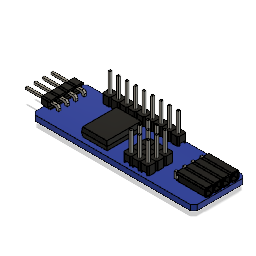
IOExpanderPCF8574T (Autodesk Fusion 360 design; units mm, degrees)
Autodesk Fusion 360 part; units mm, degrees
note: some values were not read from the file. Set by a fixed rule: which sketch regions a step uses.
sketch "Sketch1" plane through (0, 0, 0) normal (0, 1, 0) x (1, 0, 0) in component "PCB"
  line L0 (0, 0) -> (48.25, 0)
  line L1 (48.25, 0) -> (48.25, -15.6)
  line L2 (48.25, -15.6) -> (0, -15.6)
  line L3 (0, -15.6) -> (0, 0)
  dimension "d1" = 48.25
  dimension "d2" = 15.6
  dimension "d35" = 0
  dimension "d36" = 0
  dimension "d37" = 0
  dimension "d38" = 0
  measures "d2" distance of L0.start
extrude "Extrude1" add sketch "Sketch1" along normal blind 1.62 makes body 1 in component "PCB"
chamfer "Chamfer1" distance 1 angle 45 4 edges at (0, 0.81, 15.6) (48.25, 0.81, 15.6) (48.25, 0.81, 0) (0, 0.81, 0) on bodies 1 in component "PCB"
sketch "Sketch1 (1)" plane through (0, 1.62, 0) normal (0, 1, 0) x (-1, 0, 0) in component "PCB"
  line L0 (-1, 0) -> (0, 1)
  line L1 (0, 1) -> (0, 14.6)
  line L2 (0, 14.6) -> (-1, 15.6)
  line L3 (-1, 15.6) -> (-47.25, 15.6)
  line L4 (-47.25, 15.6) -> (-48.25, 14.6)
  line L5 (-48.25, 14.6) -> (-48.25, 1)
  line L6 (-48.25, 1) -> (-47.25, 0)
  line L7 (-47.25, 0) -> (-1, 0)
  line L8 (-3.3, 0) -> (-3.3, 3.3) construction
  line L9 (0, 3.3) -> (-3.3, 3.3) construction
  line L10 (-3.3, 3.3) -> (-3.3, 5.84) construction
  line L11 (-3.3, 5.84) -> (-3.3, 8.38) construction
  line L12 (-3.3, 8.38) -> (-3.3, 10.92) construction
  line L13 (0, 1.3) -> (-9, 1.3) construction
  line L14 (-9, 0) -> (-9, 1.3) construction
  line L15 (-9, 1.3) -> (-11.54, 1.3) construction
  line L16 (-11.54, 1.3) -> (-14.08, 1.3) construction
  line L17 (-14.08, 1.3) -> (-16.62, 1.3) construction
  line L18 (-16.62, 1.3) -> (-19.16, 1.3) construction
  line L19 (-19.16, 1.3) -> (-21.7, 1.3) construction
  line L20 (-21.7, 1.3) -> (-24.24, 1.3) construction
  line L21 (-24.24, 1.3) -> (-26.78, 1.3) construction
  line L22 (-26.78, 1.3) -> (-29.32, 1.3) construction
  line L23 (-38.35, 0) -> (-38.35, 3.3) construction
  line L24 (-48.25, 3.3) -> (-38.35, 3.3) construction
  line L25 (-38.35, 3.3) -> (-38.35, 5.84) construction
  line L26 (-38.35, 5.84) -> (-38.35, 8.38) construction
  line L27 (-38.35, 8.38) -> (-38.35, 10.92) construction
  line L28 (-32.45, 15.6) -> (-32.45, 13.4) construction
  line L29 (-48.25, 13.4) -> (-32.45, 13.4) construction
  line L30 (-32.45, 13.4) -> (-29.91, 13.4) construction
  line L31 (-29.91, 13.4) -> (-27.37, 13.4) construction
  line L32 (-27.37, 13.4) -> (-27.37, 10.86) construction
  line L33 (-27.37, 10.86) -> (-29.91, 10.86) construction
  line L34 (-29.91, 10.86) -> (-32.45, 10.86) construction
  line L35 (-32.45, 10.86) -> (-32.45, 8.32) construction
  line L36 (-32.45, 8.32) -> (-29.91, 8.32) construction
  line L37 (-29.91, 8.32) -> (-27.37, 8.32) construction
  dimension "d6" = 3.3
  dimension "d7" = 3.3
  dimension "d8" = 2.54
  dimension "d9" = 9
  dimension "d10" = 1.3
  dimension "d11" = 2.54
  dimension "d12" = 3.3
  dimension "d13" = 9.9
  dimension "d14" = 2.54
  dimension "d15" = 2.2
  dimension "d16" = 15.8
  dimension "d17" = 2.54
  measures "d12" distance of origin
hole "Hole1" at (27.37, 1.62, 8.32) at (29.91, 1.62, 8.32) at (32.45, 1.62, 8.32) at (32.45, 1.62, 10.86) at (29.91, 1.62, 10.86) at (27.37, 1.62, 10.86) at (27.37, 1.62, 13.4) at (29.91, 1.62, 13.4) at (32.45, 1.62, 13.4) at (38.35, 1.62, 10.92) at (38.35, 1.62, 8.38) at (38.35, 1.62, 5.84) at (38.35, 1.62, 3.3) at (29.32, 1.62, 1.3) at (26.78, 1.62, 1.3) at (24.24, 1.62, 1.3) at (21.7, 1.62, 1.3) at (19.16, 1.62, 1.3) at (16.62, 1.62, 1.3) at (14.08, 1.62, 1.3) at (11.54, 1.62, 1.3) at (9, 1.62, 1.3) at (3.3, 1.62, 10.92) at (3.3, 1.62, 8.38) at (3.3, 1.62, 5.84) at (3.3, 1.62, 3.3) direction (0, -1, 0) diameter 0.635 depth 9.6 tip angle 180 bodies 1 in component "PCB"
sketch "Sketch1 (2)" plane through (0, 0, 0) normal (0, 1, 0) x (1, 0, 0) in component "Pin"
  line L0 (0, 0) -> (5.08, 0)
  line L1 (5.08, 0) -> (5.08, -0.635)
  line L2 (5.08, -0.635) -> (0.635, -0.635)
  line L3 (0, -5.08) -> (0, 0)
  line L4 (0.635, -0.635) -> (0.635, -5.08)
  line L5 (0, -5.08) -> (0.635, -5.08)
  dimension "d3_1" = 5.08
  dimension "d29" = 0.635
  dimension "d30" = 5.08
  measures "d3_1" distance of L0.start
  measures "d30" distance of L0.start
extrude "Extrude1'" add sketch "Sketch1 (2)" along normal blind 0.635 separate body makes body 2 in component "Pin"
chamfer "Chamfer1'" distance 0.1905 angle 45 4 edges at (0.3175, 0.635, 5.08) (0.3175, 0, 5.08) (0.635, 0.3175, 5.08) (0, 0.3175, 5.08) on bodies 2 in component "Pin"
sketch "Sketch1 (3)" plane through (0, 0, 0) normal (0, 1, 0) x (1, 0, 0) in component "Plastic"
  line L0 (0, -0.3175) -> (2.159, -0.3175)
  line L1 (2.159, -1.0795) -> (2.159, 0.4445)
  line L2 (2.159, 0.4445) -> (2.1592, 0.9525) construction
  line L3 (2.159, -1.0795) -> (2.159, -1.5875) construction
  line L4 (2.159, 0.4445) -> (1.524, 0.4445)
  line L5 (2.159, -1.0795) -> (1.524, -1.0795)
  line L6 (1.524, -1.0795) -> (1.524, -1.5875)
  line L7 (1.524, 0.4445) -> (1.524, 0.9525)
  line L8 (1.524, 0.9525) -> (10.16, 0.9525)
  line L9 (10.16, 0.9525) -> (10.16, -1.5875)
  line L10 (1.524, -1.5875) -> (10.16, -1.5875)
  line L11 (0, 0) -> (0, -0.635) construction
  dimension "d7_1" = 2.159
  dimension "d8_1" = 1.524
  dimension "d9_1" = 0.508
  dimension "d11_1" = 0.635
  dimension "d12_1" = 8.636
  measures "d7_1" distance of L11.start
extrude "Extrude1''" add sketch "Sketch1 (3)" along normal mid plane 2.54 from surface at 0.3175 separate body makes body 3 in component "Plastic"
chamfer "Chamfer1''" distance 0.4 angle 45 4 edges at (5.842, 1.5875, -0.9525) (5.842, -0.9525, -0.9525) (5.842, 1.5875, 1.5875) (5.842, -0.9525, 1.5875) on bodies 3 in component "Plastic"
sketch "Sketch1 (4)" plane through (0, 0, 0) normal (0, 0, 1) x (1, 0, 0) in component "Pins bent female v2"
  line L0 (0, 0.3175) -> (0, 14)
other "PathPattern1" in component "Header"
sketch "Sketch1 (1) (2)" plane through (10.16, 0, 0) normal (1, 0, 0) x (0, 0, -1) in component "Plastic"
  line L0 (-1.5875, -0.5525) -> (-1.1875, -0.9525)
  line L1 (-1.1875, -0.9525) -> (0.5525, -0.9525)
  line L2 (0.5525, -0.9525) -> (0.9525, -0.5525)
  line L3 (0.9525, -0.5525) -> (0.9525, 1.1875)
  line L4 (0.9525, 1.1875) -> (0.5525, 1.5875)
  line L5 (0.5525, 1.5875) -> (-1.1875, 1.5875)
  line L6 (-1.1875, 1.5875) -> (-1.5875, 1.1875)
  line L7 (-1.5875, 1.1875) -> (-1.5875, -0.5525)
  line L8 (0.9525, 0.3175) -> (-0.3175, 0.3175) construction
  line L9 (-0.3175, 1.5875) -> (-0.3175, 0.3175) construction
  line L10 (-0.3175, 0.635) -> (0, 0.635)
  line L11 (0, 0.3175) -> (0, 0)
  line L12 (0, 0) -> (-0.635, 0)
  line L13 (-0.635, 0) -> (-0.635, 0.635)
  line L14 (0, 0.635) -> (0, 0.3175)
  line L15 (-0.635, 0.635) -> (-0.3175, 0.635)
  dimension "d24" = 0.635
  dimension "d25" = 0.635
  measures "d25" distance of L11.end
extrude "Extrude1'''" cut sketch "Sketch1 (1) (2)" against normal blind 5.5 contours L10 L11 L12 L13 L14 L15 bodies 3 in component "Plastic"
chamfer "Chamfer1'''" distance 0.6 angle 45 4 edges at (10.16, 0, 0.3175) (10.16, 0.3175, 0) (10.16, 0.635, 0.3175) (10.16, 0.3175, 0.635) on bodies 3 in component "Plastic"
sketch "Sketch1 (5)" plane through (0, 0, 0) normal (0, 1, 0) x (1, 0, 0) in component "Pin (1)"
  line L0 (11.684, 0) -> (11.684, -0.635)
  line L1 (0, -0.3175) -> (1.524, -0.3175) construction
  line L2 (1.524, 0) -> (1.524, -4.572)
  line L3 (1.524, 0) -> (11.684, 0)
  line L4 (11.684, -0.635) -> (2.159, -0.635)
  line L5 (2.159, -0.635) -> (1.524, -0.635) construction
  line L6 (2.159, -0.635) -> (2.159, -4.572)
  line L7 (2.159, -4.572) -> (1.524, -4.572)
  dimension "d3_2" = 11.684
  dimension "d19_2" = 1.524
  dimension "d20_2" = 0.635
  dimension "d21_1" = 4.572
  measures "d3_2" distance of origin
  measures "d19_2" distance of origin
extrude "Extrude1''''" add sketch "Sketch1 (5)" along normal blind 0.635 separate body makes body 4 in component "Pin (1)"
fillet "Fillet1" radius 0.75 2 edges at (2.159, 0.3175, 0.635) (1.524, 0.3175, 0) on bodies 4 in component "Pin (1)"
chamfer "Chamfer1''''" distance 0.1905 angle 45 8 edges at (11.684, 0.3175, 0.635) (11.684, 0.635, 0.3175) (11.684, 0.3175, 0) (11.684, 0, 0.3175) (2.159, 0.3175, 4.572) (1.524, 0.3175, 4.572) (1.8415, 0.635, 4.572) (1.8415, 0, 4.572) on bodies 4 in component "Pin (1)"
sketch "Sketch1 (6)" plane through (0, 0, 0) normal (0, 0, 1) x (1, 0, 0) in component "Pins bent male v10"
  line L0 (0, 0.3175) -> (0, 14)
  line L1 (1.7145, 0.1905) -> (1.7145, 0.4445)
  line L2 (1.7145, 0.3175) -> (0, 0.3175) construction
sketch "Sketch1 (7)" plane through (0, 0, 0) normal (0, 1, 0) x (1, 0, 0) in component "Plastic (1)"
  line L0 (0, -0.3175) -> (3.81, -0.3175)
  line L1 (3.81, -1.0795) -> (3.81, 0.4445)
  line L2 (3.81, 0.4445) -> (3.81, 0.9525) construction
  line L3 (3.81, -1.0795) -> (3.81, -1.5875) construction
  line L4 (3.81, 0.4445) -> (3.175, 0.4445)
  line L5 (3.81, -1.0795) -> (3.175, -1.0795)
  line L6 (3.175, -1.0795) -> (3.175, -1.5875)
  line L7 (3.175, 0.4445) -> (3.175, 0.9525)
  line L8 (3.175, 0.9525) -> (5.715, 0.9525)
  line L9 (5.715, 0.9525) -> (5.715, -1.5875)
  line L10 (3.175, -1.5875) -> (5.715, -1.5875)
  dimension "d7_2" = 3.81
  dimension "d8_2" = 1.524
  dimension "d9_2" = 0.508
  dimension "d11_2" = 0.635
  dimension "d12_2" = 2.54
  measures "d7_2" distance of origin
extrude "Extrude1'''''" add sketch "Sketch1 (7)" along normal mid plane 2.54 from surface at 0.3175 separate body makes body 5 in component "Plastic (1)"
chamfer "Chamfer1'''''" distance 0.4 angle 45 4 edges at (4.445, 1.5875, -0.9525) (4.445, -0.9525, -0.9525) (4.445, 1.5875, 1.5875) (4.445, -0.9525, 1.5875) on bodies 5 in component "Plastic (1)"
other "PathPattern2" in component "Pins bent male v10"
sketch "Sketch1 (8)" plane through (0, 0, 0) normal (0, 1, 0) x (1, 0, 0) in component "Pin (2)"
  line L0 (0, 0) -> (11.684, 0)
  line L1 (11.684, 0) -> (11.684, -0.635)
  line L2 (11.684, -0.635) -> (0, -0.635)
  line L3 (0, -0.635) -> (0, 0)
  dimension "d2_1" = 0.635
  dimension "d3_3" = 11.684
  measures "d3_3" distance of L0.start
extrude "Extrude1''''''" add sketch "Sketch1 (8)" along normal blind 0.635 separate body makes body 6 in component "Pin (2)"
chamfer "Chamfer1''''''" distance 0.1905 angle 45 8 edges at (0, 0.3175, 0.635) (0, 0.635, 0.3175) (0, 0.3175, 0) (0, 0, 0.3175) (11.684, 0.635, 0.3175) (11.684, 0.3175, 0) (11.684, 0, 0.3175) (11.684, 0.3175, 0.635) on bodies 6 in component "Pin (2)"
sketch "Sketch1 (9)" plane through (0, 0, 0) normal (0, 1, 0) x (1, 0, 0) in component "Plastic (2)"
  line L0 (0, -0.4445) -> (0, -0.1905)
  line L1 (0, -0.3175) -> (3.81, -0.3175)
  line L2 (3.81, -1.0795) -> (3.81, 0.4445)
  line L3 (0.1905, 0) -> (11.4935, 0) construction
  line L4 (3.81, 0.4445) -> (3.81, 0.9525) construction
  line L5 (3.81, -1.0795) -> (3.81, -1.5875) construction
  line L6 (3.81, 0.4445) -> (3.175, 0.4445)
  line L7 (3.81, -1.0795) -> (3.175, -1.0795)
  line L8 (3.175, -1.0795) -> (3.175, -1.5875)
  line L9 (3.175, 0.4445) -> (3.175, 0.9525)
  line L10 (3.175, 0.9525) -> (5.715, 0.9525)
  line L11 (5.715, 0.9525) -> (5.715, -1.5875)
  line L12 (3.175, -1.5875) -> (5.715, -1.5875)
  dimension "d7_3" = 3.81
  dimension "d8_3" = 1.524
  dimension "d9_3" = 0.508
  dimension "d11_3" = 0.635
  dimension "d12_3" = 2.54
  measures "d7_3" distance of origin
extrude "Extrude1'''''''" add sketch "Sketch1 (9)" along normal mid plane 2.54 from surface at 0.3175 separate body makes body 7 in component "Plastic (2)"
chamfer "Chamfer1'''''''" distance 0.4 angle 45 4 edges at (4.445, 1.5875, -0.9525) (4.445, -0.9525, -0.9525) (4.445, 1.5875, 1.5875) (4.445, -0.9525, 1.5875) on bodies 7 in component "Plastic (2)"
sketch "Sketch1 (10)" plane through (0, 0, 0) normal (0, 0, 1) x (1, 0, 0) in component "Pins straight male v6"
  line L0 (0, 0.1905) -> (0, 0.4445)
  line L1 (0, 0.3175) -> (0, 14)
other "PathPattern1'" in component "Header (2)"
sketch "Sketch1 (11)" plane through (0, 0, 0) normal (0, 1, 0) x (1, 0, 0) in component "Pin (3)"
  line L0 (0, 0) -> (11.684, 0)
  line L1 (11.684, 0) -> (11.684, -0.635)
  line L2 (11.684, -0.635) -> (0, -0.635)
  line L3 (0, -0.635) -> (0, 0)
  dimension "d2_2" = 0.635
  dimension "d3_4" = 11.684
  dimension "d31" = 0
  dimension "d32" = 0
  dimension "d33" = 0
  dimension "d34" = 0
  measures "d3_4" distance of L0.start
extrude "Extrude1''''''''" add sketch "Sketch1 (11)" along normal blind 0.635 separate body makes body 8 in component "Pin (3)"
chamfer "Chamfer1''''''''" distance 0.1905 angle 45 8 edges at (0, 0.3175, 0.635) (0, 0.635, 0.3175) (0, 0.3175, 0) (0, 0, 0.3175) (11.684, 0.635, 0.3175) (11.684, 0.3175, 0) (11.684, 0, 0.3175) (11.684, 0.3175, 0.635) on bodies 8 in component "Pin (3)"
sketch "Sketch1 (12)" plane through (0, 0, 0) normal (0, 1, 0) x (1, 0, 0) in component "Plastic (3)"
  line L0 (0, -0.4445) -> (0, -0.1905)
  line L1 (0, -0.3175) -> (3.81, -0.3175)
  line L2 (3.81, -1.0795) -> (3.81, 0.4445)
  line L3 (0.1905, 0) -> (11.4935, 0) construction
  line L4 (3.81, 0.4445) -> (3.81, 0.9525) construction
  line L5 (3.81, -1.0795) -> (3.81, -1.5875) construction
  line L6 (3.81, 0.4445) -> (3.175, 0.4445)
  line L7 (3.81, -1.0795) -> (3.175, -1.0795)
  line L8 (3.175, -1.0795) -> (3.175, -1.5875)
  line L9 (3.175, 0.4445) -> (3.175, 0.9525)
  line L10 (3.175, 0.9525) -> (5.715, 0.9525)
  line L11 (5.715, 0.9525) -> (5.715, -1.5875)
  line L12 (3.175, -1.5875) -> (5.715, -1.5875)
  dimension "d7_4" = 3.81
  dimension "d8_4" = 1.524
  dimension "d9_4" = 0.508
  dimension "d11_4" = 0.635
  dimension "d12_4" = 2.54
  measures "d7_4" distance of origin
extrude "Extrude1'''''''''" add sketch "Sketch1 (12)" along normal mid plane 2.54 from surface at 0.3175 separate body makes body 9 in component "Plastic (3)"
chamfer "Chamfer1'''''''''" distance 0.4 angle 45 4 edges at (4.445, 1.5875, -0.9525) (4.445, -0.9525, -0.9525) (4.445, 1.5875, 1.5875) (4.445, -0.9525, 1.5875) on bodies 9 in component "Plastic (3)"
sketch "Sketch1 (13)" plane through (0, 0, 0) normal (0, 0, 1) x (1, 0, 0) in component "Pins straight male v7"
  line L0 (0, 0.1905) -> (0, 0.4445)
  line L1 (0, 0.3175) -> (0, 14)
other "PathPattern1''" in component "Header (3)"
sketch "Sketch1 (14)" plane through (0, 1.62, 0) normal (0, 1, 0) x (-1, 0, 0) in component "Chip"
  circle A0 centre (-3.3, 5.84) radius 0.3175
  circle A1 centre (-3.3, 10.92) radius 0.3175
  circle A2 centre (-11.54, 1.3) radius 0.3175
  circle A3 centre (-16.62, 1.3) radius 0.3175
  circle A4 centre (-21.7, 1.3) radius 0.3175
  circle A5 centre (-26.78, 1.3) radius 0.3175
  circle A6 centre (-38.35, 3.3) radius 0.3175
  circle A7 centre (-38.35, 8.38) radius 0.3175
  circle A8 centre (-32.45, 13.4) radius 0.3175
  circle A9 centre (-27.37, 13.4) radius 0.3175
  circle A10 centre (-29.91, 10.86) radius 0.3175
  circle A11 centre (-32.45, 8.32) radius 0.3175
  circle A12 centre (-27.37, 8.32) radius 0.3175
  circle A13 centre (-29.91, 8.32) radius 0.3175
  circle A14 centre (-32.45, 10.86) radius 0.3175
  circle A15 centre (-27.37, 10.86) radius 0.3175
  circle A16 centre (-29.91, 13.4) radius 0.3175
  circle A17 centre (-38.35, 10.92) radius 0.3175
  circle A18 centre (-38.35, 5.84) radius 0.3175
  circle A19 centre (-29.32, 1.3) radius 0.3175
  circle A20 centre (-24.24, 1.3) radius 0.3175
  circle A21 centre (-19.16, 1.3) radius 0.3175
  circle A22 centre (-14.08, 1.3) radius 0.3175
  circle A23 centre (-9, 1.3) radius 0.3175
  circle A24 centre (-3.3, 8.38) radius 0.3175
  circle A25 centre (-3.3, 3.3) radius 0.3175
  line L0 (-1, 0) -> (0, 1)
  line L1 (0, 1) -> (0, 14.6)
  line L2 (0, 14.6) -> (-1, 15.6)
  line L3 (-1, 15.6) -> (-47.25, 15.6)
  line L4 (-47.25, 15.6) -> (-48.25, 14.6)
  line L5 (-48.25, 14.6) -> (-48.25, 1)
  line L6 (-48.25, 1) -> (-47.25, 0)
  line L7 (-47.25, 0) -> (-1, 0)
  line L8 (-13.5, 3.85) -> (-21.16, 3.85)
  line L9 (-21.16, 3.85) -> (-21.16, 14.35)
  line L10 (-21.16, 14.35) -> (-13.5, 14.35)
  line L11 (-13.5, 14.35) -> (-13.5, 3.85)
  line L12 (-17.33, 14.35) -> (-17.33, 15.6) construction
  line L13 (0, 14.35) -> (-13.5, 14.35) construction
  dimension "d111" = 7.66
  dimension "d112" = 10.5
  dimension "d113" = 1.25
  dimension "d114" = 13.5
extrude "Extrude1''''''''''" add sketch "Sketch1 (14)" along normal blind 2.6 separate body contours L8 L9 L10 L11 makes body 10 in component "Chip"
chamfer "Chamfer1''''''''''" distance 0.2 distance2 1.3 8 edges at (13.5, 4.22, 9.1) (13.5, 1.62, 9.1) (17.33, 4.22, 14.35) (17.33, 1.62, 14.35) (21.16, 4.22, 9.1) (21.16, 1.62, 9.1) (17.33, 4.22, 3.85) (17.33, 1.62, 3.85) measured on face at (16.0533, 4.22, 7.35) measured on face at (16.0533, 1.62, 7.35) measured on face at (16.0533, 4.22, 7.35) measured on face at (16.0533, 1.62, 7.35) measured on face at (16.0533, 4.22, 7.35) measured on face at (16.0533, 1.62, 7.35) measured on face at (16.0533, 4.22, 7.35) measured on face at (16.0533, 1.62, 7.35) on bodies 10 in component "Chip"
component "IO Expander PCF8574T" placed x (1, 0, 0) y (0, 1, 0) z (0, 0, 1) at (0, 0, 0)
component "PCB" placed x (1, 0, 0) y (0, 1, 0) z (0, 0, 1) at (0, 0, 0) in component "IO Expander PCF8574T"
component "Pins bent female v2" placed x (1, 0, 0) y (0, 0, 1) z (0, -1, 0) at (38.0325, 3.525, 2.9825) in component "IO Expander PCF8574T"
component "Pins bent male v10" placed x (-1, 0, 0) y (0, 0, -1) z (0, -1, 0) at (5.1415, 3.017, 11.2375) in component "IO Expander PCF8574T"
component "Pins straight male v6" placed x (0, 1, 0) y (0, 0, -1) z (-1, 0, 0) at (27.6875, -1.555, 13.7175) in component "IO Expander PCF8574T"
component "Pins straight male v6" placed x (0, 1, 0) y (0, 0, -1) z (-1, 0, 0) at (30.2275, -1.555, 13.7175) in component "IO Expander PCF8574T"
component "Pins straight male v6" placed x (0, 1, 0) y (0, 0, -1) z (-1, 0, 0) at (32.7675, -1.555, 13.7175) in component "IO Expander PCF8574T"
component "Pins straight male v7" placed x (0, 1, 0) y (-1, 0, 0) z (0, 0, 1) at (29.6375, -1.555, 0.9825) in component "IO Expander PCF8574T"
component "Chip" placed x (1, 0, 0) y (0, 1, 0) z (0, 0, 1) at (0, 0, 0) in component "IO Expander PCF8574T"
component "Header" placed x (1, 0, 0) y (0, 1, 0) z (0, 0, 1) at (0, 0, 0) in component "Pins bent female v2"
component "Header" placed x (1, 0, 0) y (0, 1, 0) z (0, 0, 1) at (0, 2.54, 0) in component "Pins bent female v2"
component "Header" placed x (1, 0, 0) y (0, 1, 0) z (0, 0, 1) at (0, 5.08, 0) in component "Pins bent female v2"
component "Header" placed x (1, 0, 0) y (0, 1, 0) z (0, 0, 1) at (0, 7.62, 0) in component "Pins bent female v2"
component "Pin" placed x (1, 0, 0) y (0, 1, 0) z (0, 0, 1) at (0, 0, 0) in component "Header"
component "Plastic" placed x (1, 0, 0) y (0, 1, 0) z (0, 0, 1) at (0, 0, 0) in component "Header"
component "Header (1)" placed x (1, 0, 0) y (0, 1, 0) z (0, 0, 1) at (0, 0, 0) in component "Pins bent male v10"
component "Header (1)" placed x (1, 0, 0) y (0, 1, 0) z (0, 0, 1) at (0, 2.54, 0) in component "Pins bent male v10"
component "Header (1)" placed x (1, 0, 0) y (0, 1, 0) z (0, 0, 1) at (0, 5.08, 0) in component "Pins bent male v10"
component "Header (1)" placed x (1, 0, 0) y (0, 1, 0) z (0, 0, 1) at (0, 7.62, 0) in component "Pins bent male v10"
component "Pin (1)" placed x (1, 0, 0) y (0, 1, 0) z (0, 0, 1) at (0, 0, 0) in component "Header (1)"
component "Plastic (1)" placed x (1, 0, 0) y (0, 1, 0) z (0, 0, 1) at (0, 0, 0) in component "Header (1)"
component "Header (2)" placed x (1, 0, 0) y (0, 1, 0) z (0, 0, 1) at (0, 0, 0) in component "Pins straight male v6"
component "Header (2)" placed x (1, 0, 0) y (0, 1, 0) z (0, 0, 1) at (0, 2.54, 0) in component "Pins straight male v6"
component "Header (2)" placed x (1, 0, 0) y (0, 1, 0) z (0, 0, 1) at (0, 5.08, 0) in component "Pins straight male v6"
component "Pin (2)" placed x (1, 0, 0) y (0, 1, 0) z (0, 0, 1) at (0, 0, 0) in component "Header (2)"
component "Plastic (2)" placed x (1, 0, 0) y (0, 1, 0) z (0, 0, 1) at (0, 0, 0) in component "Header (2)"
component "Header (3)" placed x (1, 0, 0) y (0, 1, 0) z (0, 0, 1) at (0, 0, 0) in component "Pins straight male v7"
component "Header (3)" placed x (1, 0, 0) y (0, 1, 0) z (0, 0, 1) at (0, 2.54, 0) in component "Pins straight male v7"
component "Header (3)" placed x (1, 0, 0) y (0, 1, 0) z (0, 0, 1) at (0, 5.08, 0) in component "Pins straight male v7"
component "Header (3)" placed x (1, 0, 0) y (0, 1, 0) z (0, 0, 1) at (0, 7.62, 0) in component "Pins straight male v7"
component "Header (3)" placed x (1, 0, 0) y (0, 1, 0) z (0, 0, 1) at (0, 10.16, 0) in component "Pins straight male v7"
component "Header (3)" placed x (1, 0, 0) y (0, 1, 0) z (0, 0, 1) at (0, 12.7, 0) in component "Pins straight male v7"
component "Header (3)" placed x (1, 0, 0) y (0, 1, 0) z (0, 0, 1) at (0, 15.24, 0) in component "Pins straight male v7"
component "Header (3)" placed x (1, 0, 0) y (0, 1, 0) z (0, 0, 1) at (0, 17.78, 0) in component "Pins straight male v7"
component "Header (3)" placed x (1, 0, 0) y (0, 1, 0) z (0, 0, 1) at (0, 20.32, 0) in component "Pins straight male v7"
component "Pin (3)" placed x (1, 0, 0) y (0, 1, 0) z (0, 0, 1) at (0, 0, 0) in component "Header (3)"
component "Plastic (3)" placed x (1, 0, 0) y (0, 1, 0) z (0, 0, 1) at (0, 0, 0) in component "Header (3)"
equation "pinCount = 4"
equation "d12_1 = plasticHeight"
equation "d13_1 = 0.025 in / 2"
equation "d19_1 = pinCount"
equation "d21 = pinCount"
equation "plasticHeight = 0.34 in"
equation "pinCount_1 = 4"
equation "pinCount_2 = 4"
equation "d13_2 = 0.025 in / 2"
equation "d23 = pinCount_2"
equation "pinCount_3 = 3"
equation "d13_3 = 0.025 in / 2"
equation "d19_3 = pinCount_3"
equation "d21_2 = pinCount_3"
equation "pinCount_4 = 9"
equation "d13_4 = 0.025 in / 2"
equation "d19_4 = pinCount_4"
equation "d21_3 = pinCount_4"
